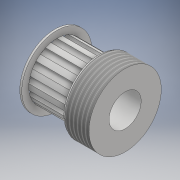
# Autodesk Inventor part: pignon 15 dents
Saved by Autodesk Inventor 2018.1 (Build 221171000, 171)
## iProperties
Created: 2022-06-29
Part Number: pignon 15 dents
Material: Generic
Document SubType Name: Modeling
Designer: Bureau
Density: 1 g/cm^3
Appearance: Default
Author: Bureau
Autodesk Inventor part; units mm, degrees
ref_plane "YZ Plane" through (0, 0, 0) normal (1, 0, 0) x (0, 1, 0)
ref_plane "XZ Plane" through (0, 0, 0) normal (0, 1, 0) x (-1, 0, 0)
ref_plane "XY Plane" through (0, 0, 0) normal (0, 0, 1) x (1, 0, 0)
sketch "Sketch1" plane through (0, 0, 0) normal (0, 0, 1) x (1, 0, 0)
  line L0 (0, 0) -> (10, 0)
  line L1 (0, 0) -> (0, 4)
  line L2 (0, 4) -> (0, 7)
  line L3 (0.5, 7) -> (11, 7)
  line L4 (11, 7) -> (11, 8.75)
  line L5 (11, 8.75) -> (11.5, 8.75)
  line L6 (17.5, 9) -> (17.5, 4)
  line L7 (17.5, 4) -> (0, 4)
  line L8 (0, 7) -> (0, 8.75)
  line L9 (0, 8.75) -> (0.5, 8.75)
  line L10 (0.5, 8.75) -> (0.5, 7)
  line L11 (17.5, 4) -> (17.5, 9)
  line L12 (17.5, 9) -> (11.5, 9)
  line L13 (11.5, 9) -> (11.5, 8.75)
  dimension "d0" = 10
  dimension "d1" = 4
  dimension "d2" = 3
  dimension "d3" = 11
  dimension "d4" = 1.75
  dimension "d6" = 9
  dimension "d8" = 0.5
  dimension "d18" = 5
  dimension "d19" = 6
  constraints: 28 end point, 9 perpendicular, 2 vertical, 1 horizontal, 1 point on line
  measures "d0" distance of L0.start L0.end
  measures "d1" distance of L0.start L1.end
  measures "d2" distance of L1.end L2.end
  measures "d3" distance of L2.end L3.end
  measures "d4" distance of L3.end L4.end
  measures "d6" vertical distance of L0.end L6.start
  measures "d8" distance of L8.end L9.end
  measures "d18" distance of L6.start L6.end
  measures "d19" distance of L6.start L12.end
revolve "Revolution1" add sketch "Sketch1" angle 360 about axis through (0, 0, 0) along (1, 0, 0)
sketch "Sketch3" plane through (0, 0, 0) normal (-1, 0, 0) x (0, 0, 1)
  arc A0 (0.7489, 6.9598) -> (-0.7489, 6.9598) centre (0, 0) ccw
  arc A1 (-0.7489, 6.9598) -> (0.7489, 6.9598) centre (0, 7) ccw
  arc A2 (-3.515, 6.0535) -> (-2.1466, 6.6627) centre (-2.8472, 6.3948) ccw
  arc A3 (-2.1466, 6.6627) -> (-3.515, 6.0535) centre (0, 0) ccw
  arc A4 (-5.6733, 4.1005) -> (-4.671, 5.2136) centre (-5.202, 4.6839) ccw
  arc A5 (-4.671, 5.2136) -> (-5.6733, 4.1005) centre (0, 0) ccw
  arc A6 (-6.8506, 1.4384) -> (-6.3878, 2.863) centre (-6.6574, 2.1631) ccw
  arc A7 (-6.3878, 2.863) -> (-6.8506, 1.4384) centre (0, 0) ccw
  arc A8 (-6.8434, -1.4723) -> (-7, 0.0173) centre (-6.9617, -0.7317) ccw
  arc A9 (-7, 0.0173) -> (-6.8434, -1.4723) centre (0, 0) ccw
  arc A10 (-5.6529, -4.1285) -> (-6.4018, -2.8313) centre (-6.0622, -3.5) ccw
  arc A11 (-6.4018, -2.8313) -> (-5.6529, -4.1285) centre (0, 0) ccw
  arc A12 (-3.485, -6.0708) -> (-4.6968, -5.1904) centre (-4.1145, -5.6631) ccw
  arc A13 (-4.6968, -5.1904) -> (-3.485, -6.0708) centre (0, 0) ccw
  arc A14 (-0.7145, -6.9634) -> (-2.1796, -6.652) centre (-1.4554, -6.847) ccw
  arc A15 (-2.1796, -6.652) -> (-0.7145, -6.9634) centre (0, 0) ccw
  arc A16 (2.1796, -6.652) -> (0.7145, -6.9634) centre (1.4554, -6.847) ccw
  arc A17 (0.7145, -6.9634) -> (2.1796, -6.652) centre (0, 0) ccw
  arc A18 (4.6968, -5.1904) -> (3.485, -6.0708) centre (4.1145, -5.6631) ccw
  arc A19 (3.485, -6.0708) -> (4.6968, -5.1904) centre (0, 0) ccw
  arc A20 (6.4018, -2.8313) -> (5.6529, -4.1285) centre (6.0622, -3.5) ccw
  arc A21 (5.6529, -4.1285) -> (6.4018, -2.8313) centre (0, 0) ccw
  arc A22 (7, 0.0173) -> (6.8434, -1.4723) centre (6.9617, -0.7317) ccw
  arc A23 (6.8434, -1.4723) -> (7, 0.0173) centre (0, 0) ccw
  arc A24 (6.3878, 2.863) -> (6.8506, 1.4384) centre (6.6574, 2.1631) ccw
  arc A25 (6.8506, 1.4384) -> (6.3878, 2.863) centre (0, 0) ccw
  arc A26 (4.671, 5.2136) -> (5.6733, 4.1005) centre (5.202, 4.6839) ccw
  arc A27 (5.6733, 4.1005) -> (4.671, 5.2136) centre (0, 0) ccw
  arc A28 (2.1466, 6.6627) -> (3.515, 6.0535) centre (2.8472, 6.3948) ccw
  arc A29 (3.515, 6.0535) -> (2.1466, 6.6627) centre (0, 0) ccw
  dimension "d10" = 14
  dimension "d11" = 1.5
  dimension "d14" = 360
  constraints: 75 point on circle, 30 centre point, 1 coincident, 91 other
  measures "d10" diameter of A0
  measures "d11" diameter of A1
extrude "Extrusion1" cut sketch "Sketch3" against normal blind 11
thread "Thread1" size "M16x1" class "6g" standard "ANSI Metric M Profile" full length
body "Solid1"
